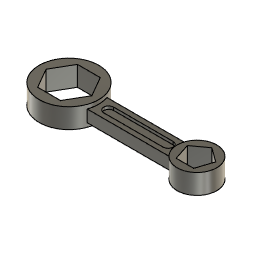
e2 (Autodesk Fusion 360 design; units mm, degrees)
Autodesk Fusion 360 part; units mm, degrees
sketch "Sketch1" plane through (0, 0, 0) normal (0, 0, 1) x (1, 0, 0)
  circle A0 centre (0, 0) radius 30
  circle A1 centre (129, 0) radius 20
  line L0 (129, 15) -> (114.7342, 4.6353)
  line L1 (114.7342, 4.6353) -> (120.1832, -12.1353)
  line L2 (120.1832, -12.1353) -> (137.8168, -12.1353)
  line L3 (137.8168, -12.1353) -> (143.2658, 4.6353)
  line L4 (143.2658, 4.6353) -> (129, 15)
  line L5 (-11.547, 20) -> (-23.094, 0)
  line L6 (-23.094, 0) -> (-11.547, -20)
  line L7 (-11.547, -20) -> (11.547, -20)
  line L8 (11.547, -20) -> (23.094, 0)
  line L9 (23.094, 0) -> (11.547, 20)
  line L10 (11.547, 20) -> (-11.547, 20)
  line L11 (28.2843, 10) -> (111.6795, 10)
  line L12 (28.2843, -10) -> (111.6795, -10)
  line L13 (100, 5) -> (40, 5)
  line L14 (40, -5) -> (100, -5)
  line L15 (105, 5) -> (35, -5) construction
  line L16 (35, 5) -> (105, -5) construction
  arc A2 (40, 5) -> (40, -5) centre (40, 0) ccw
  arc A3 (100, -5) -> (100, 5) centre (100, 0) ccw
  point P0 (129, 0)
  point P1 (70, 0)
  dimension "d6" = 129
  dimension "d9" = 20
  dimension "d10" = 60
  dimension "d11" = 40
  dimension "d12" = 15
  dimension "d17" = 70
  dimension "d18" = 10
  constraint coincident A0.centre origin
  constraint coincident P0 A1.centre
  constraint horizontal L12
  constraint horizontal L13
  constraint parallel L13 L14
  constraint coincident L15 P1
  constraint coincident L16 P1
  constraint tangent L13 A3
  constraint tangent L14 A3
  constraint tangent L14 A2
  constraint tangent L13 A2
  constraint coincident A1 L12.end
  constraint coincident A1 L11.end
  constraint coincident A0 L11.start
  constraint coincident A0 L12.start
  measures "d6" distance of A0.centre A1.centre
  measures "d9" distance of A0.centre L10
  measures "d10" diameter of A0
  measures "d11" diameter of A1
  measures "d12" distance of L0.start P0
  measures "d17" distance of L15.end L16.end
  measures "d18" distance of L16.start L15.end
extrude "Extrude1" add sketch "Sketch1" along normal mid plane 20 contours A0 | A1 makes body 1 at (27.1662, -12.7278, 3.3333) makes body 2 at (148.9006, -1.9914, -3.3333)
extrude "Extrude2" add sketch "Sketch1" along normal mid plane 12 contours A0 A1 L11 L12 bodies 1 2
extrude "Extrude3" add sketch "Sketch1" along normal blind 3 contours L13 L14 A2 A3 bodies 1
